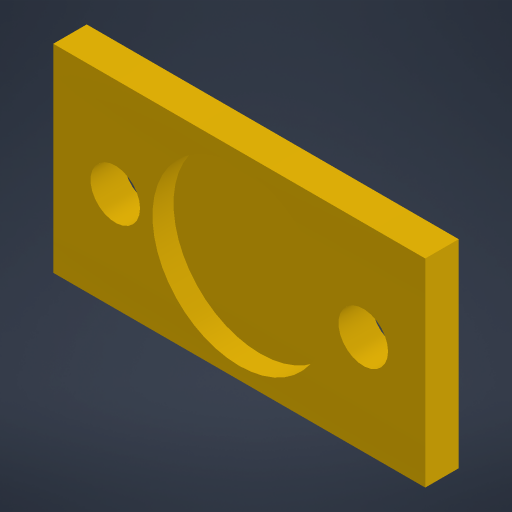
# Autodesk Inventor part: AxleCovers
Saved by Autodesk Inventor 2024.2 (Build 282272000, 272)
## iProperties
Created: 2023-09-28
Part Number: AxleCovers
Material: Generic
Document SubType Name: Modeling
Designer: tech
Density: 1 g/cm^3
Appearance: Default
Author: tech
Autodesk Inventor part; units mm, degrees
ref_plane "YZ Plane" through (0, 0, 0) normal (1, 0, 0) x (0, 1, 0)
ref_plane "XZ Plane" through (0, 0, 0) normal (0, 1, 0) x (-1, 0, 0)
ref_plane "XY Plane" through (0, 0, 0) normal (0, 0, 1) x (1, 0, 0)
sketch "Sketch6" plane through (0, 0, 0) normal (0, 0, 1) x (1, 0, 0)
  circle A0 centre (0, 0) radius 7.62
  circle A1 centre (0, 0) radius 8.89
  line L0 (0, 8.89) -> (-19.05, 8.89)
  line L1 (-19.05, 8.89) -> (-19.05, -8.89)
  line L2 (-19.05, -8.89) -> (19.05, -8.89)
  line L3 (19.05, -8.89) -> (19.05, 8.89)
  line L4 (19.05, 8.89) -> (0, 8.89)
  circle A2 centre (-12.7, 0) radius 2.537
  circle A3 centre (12.7, 0) radius 2.54
  point P0 (0, -8.89)
  dimension "d23" = 17.78
  dimension "d22" = 15.24
  dimension "d24" = 19.05
  dimension "d25" = 38.1
  dimension "d26" = 5.08
  constraints: 10 end point, 3 centre point, 3 perpendicular, 2 coincident, 2 horizontal, 1 point on line, 3 other
  measures "d22" diameter of A0
  measures "d24" distance of L0.start L0.end
  measures "d25" distance of L1.end L2.end
  measures "d26" diameter of A3
extrude "Extrusion6" add sketch "Sketch6" along normal blind 2.159 contours A1 L4 L3 L2 | A1 L2 L1 L0
extrude "Extrusion7" add sketch "Sketch6" against normal blind 1.27 contours A0 | A1 | A1 L4 L3 L2 | A1 L2 L1 L0
sketch "Sketch7" plane through (-19.05, 8.89, 2.159) normal (0, 1, 0) x (1, 0, 0)
  line L0 (19.05, 0) -> (0, 0) projected
  line L1 (0, 3.429) -> (0, 0) projected
  line L2 (0, 0) -> (0, 3.429)
  line L3 (38.1, 3.429) -> (38.1, 0) projected
  line L4 (0, 3.429) -> (38.1, 3.429)
  line L5 (38.1, 3.429) -> (38.1, 0)
  line L6 (38.1, 0) -> (0, 0)
  point P0 (19.05, 2.159)
  constraints: 8 end point, 2 perpendicular, 1 collinear, 1 vertical
extrude "Extrusion8" add sketch "Sketch7" along normal blind 1.27
sketch "Sketch8" plane through (-19.05, -8.89, 2.159) normal (0, -1, 0) x (1, 0, 0)
  line L0 (38.1, -3.429) -> (0, -3.429) projected
  line L1 (0, 0) -> (0, -3.429) projected
  line L2 (0, -3.429) -> (0, 0)
  line L3 (19.05, 0) -> (38.1, 0) projected
  line L4 (0, 0) -> (38.1, 0)
  line L5 (38.1, -3.429) -> (38.1, 0) projected
  line L6 (38.1, 0) -> (38.1, -3.429)
  line L7 (38.1, -3.429) -> (0, -3.429)
  point P0 (19.05, -2.159)
  constraints: 8 end point, 2 collinear, 1 perpendicular, 1 vertical
extrude "Extrusion9" add sketch "Sketch8" along normal blind 1.27
body "Solid2"
